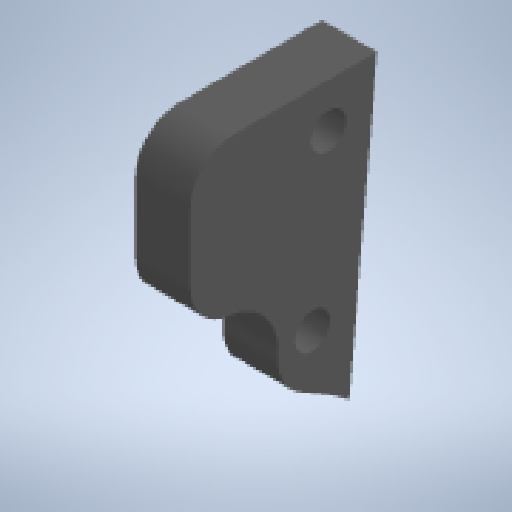
# Autodesk Inventor part: toe_springjoint_cover_upper_left
Saved by Autodesk Inventor 2024.1 (Build 281209000, 209)
## iProperties
Created: 2024-02-25
Part Number: toe_springjoint_cover_upper_left
Material: 一般
Document SubType Name: Modeling
Designer: hibik
Density: 1 g/cm^3
Appearance: 既定
Author: hibik
Autodesk Inventor part; units mm, degrees
ref_plane "YZ Plane" through (0, 0, 0) normal (1, 0, 0) x (0, 1, 0)
ref_plane "XZ Plane" through (0, 0, 0) normal (0, 1, 0) x (-1, 0, 0)
ref_plane "XY Plane" through (0, 0, 0) normal (0, 0, 1) x (1, 0, 0)
sketch "スケッチ1" plane through (0, 0, 0) normal (1, 0, 0) x (0, 1, 0)
  circle A0 centre (0, 0) radius 9
  line L0 (50, 5.5) -> (-9, 5.5)
  line L1 (-9, 5.5) -> (-9, -13.5)
  line L2 (-9, -13.5) -> (50, -13.5)
  line L3 (50, -13.5) -> (50, 5.5)
  line L4 (50, 13.5) -> (-9, 13.5)
  line L5 (-9, 13.5) -> (-9, -13.5)
  line L6 (-9, -13.5) -> (50, -13.5)
  line L7 (50, -13.5) -> (50, 13.5)
  line L8 (-20.8, 0) -> (61.8, 0) projected
  point P0 (-9, 0)
  dimension "d0" = 18
  dimension "d3" = 19
  dimension "d4" = 27
  constraints: 16 end point, 4 parallel, 2 horizontal, 2 perpendicular, 1 centre point, 1 coincident, 1 midpoint, 1 point on line, 1 tangent
  measures "d0" diameter of A0
  measures "d3" distance of L2.end L0.start
  measures "d4" distance of L4.end L1.end
extrude "押し出し1" add sketch "スケッチ1" along normal blind 1.5 contours L8 L3 L2 L1 A0 | A0 L0 L3 L8 | L1 L0 A0
sketch "スケッチ2" plane through (0, 0, 0) normal (-1, 0, 0) x (0, 0, 1)
  arc A0 (-0.2778, 12.9845) -> (-2.4907, 10.2851) centre (0, 10.5) ccw projected
  line L0 (-3.4833, 8.3812) -> (-3.5, 8.3716) projected
  line L1 (-3.5, 8.3716) -> (-3.5, 20) projected
  line L2 (-3.5, 20) -> (-0.5, 20) projected
  line L3 (-7, 20) -> (-3.5, 20) projected
  arc A1 (-4.5, 7.7942) -> (-5.7273, 6.9425) centre (0, 0) ccw projected
  line L4 (-3.5, 8.3716) -> (-4.5, 7.7942) projected
  arc A2 (5.5, 7.1239) -> (0, -9) centre (0, 0) ccw projected
  line L5 (5.5, 50) -> (5.5, 7.1239) projected
  line L6 (-13.5, 50) -> (5.5, 50) projected
  line L7 (-13.5, -9) -> (-13.5, 50) projected
  line L8 (0, -9) -> (-13.5, -9) projected
  line L9 (5.5, -9) -> (0, -9) projected
  line L10 (5.5, -7.1239) -> (5.5, -9) projected
  arc A3 (0, -9) -> (5.5, -7.1239) centre (0, 0) ccw projected
  arc A4 (-3.4833, 8.3812) -> (-2.4907, 10.2851) centre (-4.4833, 10.1132) ccw projected
  arc A5 (1.5, 18) -> (-0.5, 20) centre (-0.5, 18) ccw projected
  line L11 (1.5, 18) -> (1.5, 14.9721) projected
  arc A6 (-0.2778, 12.9845) -> (1.5, 14.9721) centre (-0.5, 14.9721) ccw projected
  line L12 (-9, 8.4853) -> (-9, 18) projected
  arc A7 (-7, 20) -> (-9, 18) centre (-7, 18) ccw projected
  arc A8 (-9, 8.4853) -> (-5.7273, 6.9425) centre (-7, 8.4853) ccw projected
  point P0 (-4.5, 7.7942)
  point P1 (-5.7273, 6.9425)
extrude "押し出し2" cut sketch "スケッチ2" against normal through all contours A6 L11 A5 L2 L3 A7 L12 A8 A2 L8 L7 L6 L5 L4 L0 A4 A0 | A3 L10 L9
sketch "スケッチ3" plane through (0, 0, 0) normal (-1, 0, 0) x (0, 0, 1)
  line L0 (-3.5, 20) -> (-3.5, 8.3716) projected
  line L1 (-4.5, 7.7942) -> (-3.4833, 8.3812) projected
  arc A0 (-0.2778, 12.9845) -> (-2.4907, 10.2851) centre (0, 10.5) ccw projected
  line L2 (-0.5, 20) -> (-7, 20) projected
  arc A1 (-4.5, 7.7942) -> (-5.7273, 6.9425) centre (0, 0) ccw projected
  line L3 (-3.5, 20) -> (-2.5, 20)
  line L4 (-2.5, 20) -> (-2.5, 8.3716)
  line L5 (-2.5, 8.3716) -> (-3.5, 8.3716)
  line L6 (-3.5, 8.3716) -> (-3.5, 20)
  arc A2 (-3.4833, 8.3812) -> (-2.4907, 10.2851) centre (-4.4833, 10.1132) ccw projected
  arc A3 (-0.2778, 12.9845) -> (1.5, 14.9721) centre (-0.5, 14.9721) ccw projected
  line L7 (1.5, 14.9721) -> (1.5, 18) projected
  arc A4 (1.5, 18) -> (-0.5, 20) centre (-0.5, 18) ccw projected
  arc A5 (-7, 20) -> (-9, 18) centre (-7, 18) ccw projected
  line L8 (-9, 18) -> (-9, 8.4853) projected
  arc A6 (-9, 8.4853) -> (-5.7273, 6.9425) centre (-7, 8.4853) ccw projected
  line L9 (-2.5, 8.3716) -> (-2.5, 10.5)
  point P0 (-2.5, 9.8557)
  dimension "d7" = 1
  constraints: 10 end point, 2 parallel, 1 horizontal, 1 perpendicular, 1 point on circle, 1 point on line, 1 vertical
  measures "d7" distance between parallel lines of L4 L0
extrude "押し出し3" add sketch "スケッチ3" along normal blind 1 contours L2 A4 L7 A3 A0 L4 | A0 A2 L4
sketch "スケッチ4" plane through (1.5, 0, 0) normal (1, 0, 0) x (0, 0, -1)
  circle A0 centre (7, 18) radius 0.8
  circle A1 centre (7, 10.5) radius 0.8
  line L0 (7, 20) -> (0.5, 20) projected
  arc A2 (2.4907, 10.2851) -> (0.2778, 12.9845) centre (0, 10.5) ccw projected
  point P0 (0, 0)
  point P1 (-1.5, 20)
  point P2 (-1.5, 12.5)
  point P3 (2.1169, 9.1701)
  dimension "d10" = 1.6
  dimension "d11" = 1.6
  dimension "d12" = 2
  constraints: 2 centre point, 2 vertical alignment, 1 horizontal alignment
  measures "d10" diameter of A0
  measures "d11" diameter of A1
  measures "d12" distance from line of L0 A0.centre
extrude "押し出し4" cut sketch "スケッチ4" against normal through all
